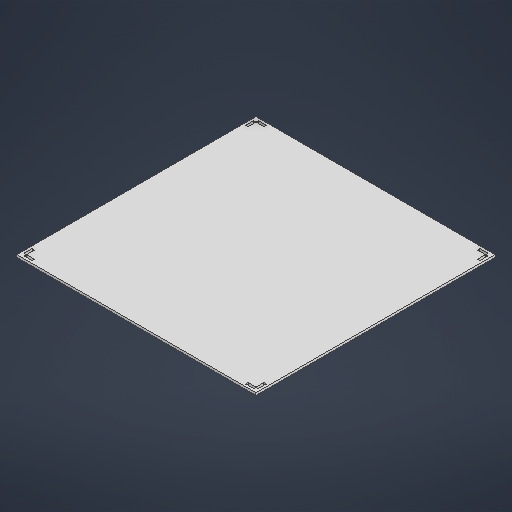
# Autodesk Inventor part: Base_de_equipo
Saved by Autodesk Inventor 2026 (Build 300175000, 175)
## iProperties
Created: 2026-05-15
Part Number: Base_de_equipo
Material: Generic
Document SubType Name: Modeling
Designer: juana
Density: 1 g/cm^3
Appearance: Default
Author: juana
Autodesk Inventor part; units mm, degrees
ref_plane "YZ Plane" through (0, 0, 0) normal (1, 0, 0) x (0, 1, 0)
ref_plane "XZ Plane" through (0, 0, 0) normal (0, 1, 0) x (-1, 0, 0)
ref_plane "XY Plane" through (0, 0, 0) normal (0, 0, 1) x (1, 0, 0)
sketch "Sketch1" plane through (0, 0, 0) normal (0, 1, 0) x (-1, 0, 0)
  line L0 (0, -300) -> (-300, -300)
  line L1 (-300, -300) -> (-300, 0)
  line L2 (-300, 0) -> (0, 0)
  line L3 (0, 0) -> (0, -300)
  dimension "d0" = 300
  dimension "d1" = 300
  constraints: 8 end point, 2 parallel, 1 coincident, 1 horizontal, 1 horizontal alignment, 1 perpendicular
  measures "d0" distance of L2.end L0.start
  measures "d1" distance of L0.start L0.end
extrude "Extrusion1" add sketch "Sketch1" along normal blind 3
sketch "Sketch2" plane through (0, 3, 0) normal (0, 1, 0) x (1, 0, 0)
  line L0 (6, 3) -> (16, 3)
  line L1 (16, 3) -> (16, 6)
  line L2 (16, 6) -> (6, 6)
  line L3 (6, 6) -> (6, 3)
  line L4 (6, 6) -> (3, 6)
  line L5 (3, 6) -> (3, 16)
  line L6 (3, 16) -> (6, 16)
  line L7 (6, 16) -> (6, 6)
  line L8 (0, 0) -> (300, 0) construction
  line L9 (0, 300) -> (0, 0) construction
  line L10 (150, 0) -> (150, 300) construction
  line L11 (300, 300) -> (0, 300) construction
  line L12 (0, 150) -> (300, 150) construction
  line L13 (300, 0) -> (300, 300) construction
  line L14 (294, 3) -> (284, 3)
  line L15 (284, 3) -> (284, 6)
  line L16 (284, 6) -> (294, 6)
  line L17 (294, 6) -> (294, 3)
  line L18 (294, 6) -> (297, 6)
  line L19 (297, 6) -> (297, 16)
  line L20 (297, 16) -> (294, 16)
  line L21 (294, 16) -> (294, 6)
  line L22 (6, 297) -> (16, 297)
  line L23 (16, 297) -> (16, 294)
  line L24 (16, 294) -> (6, 294)
  line L25 (6, 294) -> (6, 297)
  line L26 (6, 294) -> (3, 294)
  line L27 (3, 294) -> (3, 284)
  line L28 (3, 284) -> (6, 284)
  line L29 (6, 284) -> (6, 294)
  line L30 (294, 294) -> (294, 297)
  line L31 (294, 297) -> (284, 297)
  line L32 (284, 297) -> (284, 294)
  line L33 (284, 294) -> (294, 294)
  line L34 (297, 294) -> (297, 284)
  line L35 (297, 284) -> (294, 284)
  line L36 (294, 284) -> (294, 294)
  line L37 (294, 294) -> (297, 294)
  dimension "d4" = 10
  dimension "d5" = 3
  dimension "d6" = 6
  dimension "d7" = 3
  dimension "d8" = 3
  dimension "d9" = 10
  constraints: 68 end point, 21 symmetric about line, 4 midpoint, 4 parallel, 2 horizontal, 2 perpendicular
  measures "d4" distance of L1.end L2.end
  measures "d5" distance of L2.end L0.start
  measures "d6" distance from line of L8.start L3
  measures "d7" distance from line of L8.start L0
  measures "d8" distance of L2.end L4.end
  measures "d9" distance of L4.end L5.end
extrude "Extrusion2" cut sketch "Sketch2" against normal blind 10
equation "\"d10\" = d4"
body "Solid1"
